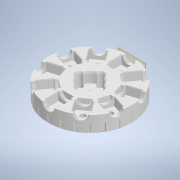
# Autodesk Inventor part: tool_adapter
Saved by Autodesk Inventor 2021 (Build 250183000, 183)
## iProperties
Created: 2021-02-06
Part Number: tool_adapter
Material: Generic
Document SubType Name: Modeling
Designer: dsdan
Density: 1 g/cm^3
Appearance: Default
Author: dsdan
Autodesk Inventor part; units mm, degrees
ref_plane "YZ Plane" through (0, 0, 0) normal (1, 0, 0) x (0, 1, 0)
ref_plane "XZ Plane" through (0, 0, 0) normal (0, 1, 0) x (-1, 0, 0)
sketch "Sketch12" plane through (0, 0, 0) normal (0, -1, 0) x (1, 0, 0)
  line L0 (-15.4337, -47.5) -> (15.4337, -47.5)
  circle A0 centre (0, -37.5) radius 3.25
  arc A1 (-15.4337, -47.5) -> (15.4337, -47.5) centre (0, 0) ccw
  line L1 (-15.4337, -47.5) -> (0, 0)
  line L2 (0, 0) -> (15.4337, -47.5)
  dimension "d60" = 6.5
  dimension "d61" = 10
  dimension "d104" = 36
  dimension "d106" = 37.5
  constraints: 6 end point, 2 centre point, 2 point on circle, 1 coincident, 1 horizontal, 1 vertical alignment
  measures "d60" diameter of A0
  measures "d61" distance from line of L0 A0.centre
  measures "d104" angle of L1 L2
  measures "d106" distance of point (0, 0) A0.centre
extrude "Extrusion9" add sketch "Sketch12" against normal blind 9
sketch "Sketch17" plane through (0, 9, 0) normal (0, 1, 0) x (1, 0, 0)
  line L0 (-7.9, 45.4) -> (7.9, 45.4)
  line L1 (7.9, 45.4) -> (7.9, 29.6)
  line L2 (7.9, 29.6) -> (-7.9, 29.6)
  line L3 (-7.9, 29.6) -> (-7.9, 45.4)
  line L4 (-7.9, 45.4) -> (7.9, 29.6) construction
  line L5 (7.9, 45.4) -> (-7.9, 29.6) construction
  arc A0 (15.4337, 47.5) -> (-15.4337, 47.5) centre (0, 0) ccw projected
  line L6 (-15.4337, 47.5) -> (0, 0) projected
  line L7 (0, 0) -> (15.4337, 47.5) projected
  circle A1 centre (0, 37.5) radius 3.25 construction
  dimension "d105" = 15.8
  constraints: 12 end point, 2 midpoint, 2 parallel, 2 perpendicular, 1 coincident, 1 horizontal
  measures "d105" distance of L0.start L0.end
extrude "Extrusion13" add sketch "Sketch17" along normal blind 10
ref_plane "Work Plane6" through (0, 0, -49.9445) normal (0, 0, 1) x (1, 0, 0)
sketch "Sketch18" plane through (0, 0, -49.9445) normal (0, 0, 1) x (1, 0, 0)
  circle A0 centre (0, 19.287) radius 6.5
  line L0 (-7.9, 9) -> (7.9, 9) projected
  line L1 (7.9, 9) -> (-7.9, 9) projected
  line L2 (-3.25, 9) -> (3.25, 9) projected
  point P0 (0, 0)
  point P1 (0, 9)
  dimension "d109" = 13
  dimension "d110" = 10.287
  constraints: 1 centre point, 1 midpoint, 1 vertical alignment
  measures "d109" diameter of A0
  measures "d110" distance from line of L0 A0.centre
extrude "Extrusion14" cut sketch "Sketch18" along normal blind 24
sketch "Sketch16" plane through (0, 0, 0) normal (0, -1, 0) x (1, 0, 0)
  circle A0 centre (0, -37.5) radius 7.5
  circle A1 centre (0, -37.5) radius 3.25 projected
  point P0 (0, 0)
  dimension "d91" = 15
  constraints: 1 centre point, 1 concentric
  measures "d91" diameter of A0
extrude "Extrusion12" cut sketch "Sketch16" against normal blind 6 contours A0 | A1
chamfer "Chamfer3" distance 0.7 angle 45 10 edges at (-7.5, 0, -37.5) (-7.9, 19, -37.5) (-7.1968, 19, -29.6) (7.1968, 19, -29.6) (7.1968, 19, -45.4) (7.9, 19, -37.5) (-7.1968, 19, -45.4) (-4.8504, 14.9599, -49.7084) (4.8499, 14.9594, -49.7084) (0, 12.787, -29.6)
pattern_circular "Circular Pattern3" count 10 over 360 about axis through (0, 0, 0) along (0, 1, 0) of "Extrusion9", "Extrusion12", "Chamfer3", "Extrusion13", "Extrusion14"
sketch "Sketch2" plane through (0, 19, 0) normal (0, 1, 0) x (1, 0, 0)
  circle A0 centre (0, -12.5) radius 3.75
  circle A1 centre (12.5, 0) radius 3.75
  circle A2 centre (0, 12.5) radius 3.75
  circle A3 centre (-12.5, 0) radius 3.75
  point P0 (0, 0)
  point P1 (0, 0)
  dimension "d3" = 7.5
  dimension "d6" = 360
  dimension "d8" = 12.5
  constraints: 4 centre point, 1 coincident, 1 vertical alignment, 9 other
  measures "d3" diameter of A0
  measures "d8" distance of point (0, 0) A0.centre
extrude "Extrusion2" cut sketch "Sketch2" against normal blind 16
sketch "Sketch3" plane through (0, 3, 12.5) normal (0, 1, 0) x (1, 0, 0)
  circle A0 centre (0, 0) radius 2.05
  circle A1 centre (-12.5, 12.5) radius 2.05
  circle A2 centre (0, 25) radius 2.05
  circle A3 centre (12.5, 12.5) radius 2.05
  point P0 (0, 12.5)
  point P1 (0, 25)
  dimension "d11" = 4.1
  constraints: 4 centre point, 4 coincident, 3 equal radius
  measures "d11" diameter of A0
extrude "Extrusion3" cut sketch "Sketch3" against normal through all
sketch "Sketch4" plane through (0, 19, 0) normal (0, 1, 0) x (1, 0, 0)
  circle A0 centre (0, 0) radius 12.75
  point P0 (0, 0)
  dimension "d17" = 25.5
  constraints: 2 coincident, 1 centre point
  measures "d17" diameter of A0
extrude "Extrusion4" cut sketch "Sketch4" against normal blind 11.5
sketch "Sketch5" plane through (0, 7.5, 0) normal (0, 1, 0) x (1, 0, 0)
  circle A0 centre (0, 0) radius 2.65
  dimension "d20" = 5.3
  constraints: 1 centre point, 1 coincident
  measures "d20" diameter of A0
extrude "Extrusion5" cut sketch "Sketch5" against normal through all
chamfer "Chamfer4" distance 1 angle 45 1 edges at (-40.4059, 0, -29.3566)
sketch "Sketch14" plane through (0, 0, 0) normal (0, -1, 0) x (1, 0, 0)
  line L0 (-0.5, -49.942) -> (0, -48.942)
  line L1 (0, -48.942) -> (0.5, -49.942)
  circle A0 centre (0, 0) radius 49.9445 projected
  dimension "d70" = 1
  dimension "d71" = 0.5
  dimension "d78" = 1
  constraints: 4 end point, 2 point on circle, 1 vertical alignment
  measures "d70" distance of L1.end L0.start
  measures "d71" horizontal distance of L1.end L0.end
  measures "d78" vertical distance of L0.start L0.end
extrude "Extrusion10" cut sketch "Sketch14" against normal blind 10 contours L0 L1 A0 picked at (0.2222, -49.6094)
pattern_circular "Circular Pattern4" count 24 over 360 about axis through (0, 7.5, 0) along (0, -1, 0) of "Extrusion10"
chamfer "Chamfer5" distance 1.5 angle 45 20 edges at (3.8387, 19, -12.1584) (7.4943, 19, -10.315) (11.4082, 19, -5.6934) (3.7468, 19, -12.3449) (-0.1551, 19, -16.2468) (-3.8387, 19, -12.1584) (-7.4943, 19, -10.315) (-11.4082, 19, -5.6934) (-15.0397, 19, -2.7591) (-15.0397, 19, 2.7591) (-11.4082, 19, 5.6934) (-7.4943, 19, 10.315) (-3.8387, 19, 12.1584) (3.7468, 19, 12.3449) (-0.1551, 19, 16.2468) (11.4082, 19, 5.6934) (3.8387, 19, 12.1584) (7.4943, 19, 10.315) (15.0397, 19, -2.7591) (15.0397, 19, 2.7591)
equation "\"d71\" = 0.5 * d70"
body "Solid1"
body "Solid2"
